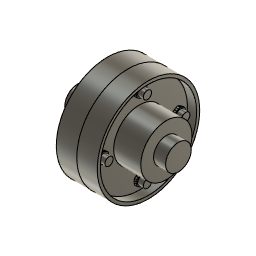
Sketch31_Final v1 (Autodesk Fusion 360 design; units mm, degrees)
Autodesk Fusion 360 part; units mm, degrees
sketch "Sketch1" plane through (0, 0, 0) normal (0, 1, 0) x (1, 0, 0)
  line L0 (0, -25) -> (0, -45)
  line L1 (0, -25) -> (0, -100)
  line L2 (0, -100) -> (40, -100)
  line L3 (40, -100) -> (40, -94)
  line L4 (0, -100) -> (22, -100)
  line L5 (22, -100) -> (22, -94)
  line L6 (22, -94) -> (0, -94)
  line L7 (40, -94) -> (22, -94)
  line L8 (0, -25) -> (0, -50)
  line L9 (22, -94) -> (22, -50)
  line L10 (0, -50) -> (22, -50)
  line L11 (75, -25) -> (75, -50)
  line L12 (22, -50) -> (75, -50)
  line L13 (0, -45) -> (-5, -45)
  line L14 (-5, -45) -> (-5, -25)
  line L15 (0, -25) -> (-5, -25)
  line L16 (0, -25) -> (75, -25)
  dimension "d3" = 45
  dimension "d4" = 100
  dimension "d5" = 40
  dimension "d6" = 6
  dimension "d9" = 25
  dimension "d10" = 50
  dimension "d12" = 5
  constraint vertical L0
  constraint parallel L0 L1
  constraint perpendicular L1 L2
  constraint perpendicular L2 L3
  constraint perpendicular L1 L4
  constraint perpendicular L4 L5
  constraint coincident L1 L6.end
  constraint perpendicular L1 L6
  constraint perpendicular L6 L9
  constraint perpendicular L9 L10
  constraint perpendicular L11 L12
  constraint perpendicular L8 L13
  constraint perpendicular L13 L14
  constraint perpendicular L14 L15
  measures "d3" distance of origin L0.end
  measures "d4" distance of origin L1.end
  measures "d5" distance of L1.end L2.end
  measures "d6" distance of L2.end L3.end
  measures "d9" distance of origin L0.start
  measures "d10" distance of origin L8.end
  measures "d12" distance of L0.end L13.end
revolve "Revolve1" add sketch "Sketch1" angle 360 about axis through (1.75, 0, 0) along (1, 0, 0) makes body 1
hole "Hole1" at (0, -2.3677, 72.2147) direction (1, 0, 0) diameter 16 depth 70 tip angle 118 bodies 1
pattern_circular "C-Pattern1" count 4 over 360 about axis through (1.75, 0, 0) along (1, 0, 0) of "Hole1"
copy_body "Body->Comp1" bodies 1 removing the originals makes body 2 in component "Male Flange"
sketch "Sketch2" plane through (0, 0, 0) normal (0, 1, 0) x (1, 0, 0)
  line L0 (5, -25) -> (75, -25)
  line L1 (75, -25) -> (75, -50)
  line L2 (75, -50) -> (0, -50)
  line L3 (0, -50) -> (0, -100)
  line L4 (0, -100) -> (40, -100)
  line L5 (40, -100) -> (40, -94)
  line L6 (40, -94) -> (22, -94)
  line L7 (22, -94) -> (22, -50)
  line L8 (0, -50) -> (0, -45)
  line L9 (5, -25) -> (5, -45)
  line L10 (5, -45) -> (0, -45)
  constraint horizontal L0
  constraint perpendicular L0 L1
  constraint perpendicular L1 L2
  constraint perpendicular L0 L3
  constraint perpendicular L3 L4
  constraint perpendicular L4 L5
  constraint perpendicular L5 L6
  constraint coincident L2 L7.end
  constraint perpendicular L2 L7
  constraint perpendicular L0 L8
  constraint perpendicular L0 L9
  constraint perpendicular L8 L10
revolve "Revolve2" add sketch "Sketch2" angle 360 about axis through (1.75, 0, 0) along (1, 0, 0) separate body makes body 3
hole "Hole2" at (0, 10.3242, 67.7446) direction (1, 0, 0) diameter 16 depth 70 tip angle 118 bodies 3
pattern_circular "C-Pattern2" count 4 over 360 about axis through (1.75, 0, 0) along (1, 0, 0) of "Hole2"
copy_body "Body->Comp2" bodies 3 removing the originals makes body 4 in component "Female Flange"
sketch "Sketch3" plane through (0, 0, 0) normal (1, 0, 0) x (0, 1, 0)
  circle A0 centre (0, 0) radius 25
  dimension "d26" = 50
  constraint coincident A0.centre origin
  measures "d26" diameter of A0
extrude "Extrude1" add sketch "Sketch3" along normal blind 100 separate body makes body 5
copy_body "Body->Comp3" bodies 5 removing the originals makes body 6 in component "Shaft"
sketch "Sketch4" plane through (0, 0, 0) normal (0, 1, 0) x (1, 0, 0)
  line L0 (0, 0) -> (0, -8)
  line L1 (0, -8) -> (44, -8)
  line L2 (44, -8) -> (44, 0)
  line L3 (44, 0) -> (0, 0)
  line L4 (0, 0) -> (0, -16)
  line L5 (0, -16) -> (-16, -16)
  line L6 (-16, -16) -> (-16, 0)
  line L7 (-16, 0) -> (0, 0)
  line L8 (0, -8) -> (60, -8)
  line L9 (60, -8) -> (60, 0)
  line L10 (60, 0) -> (44, 0)
  dimension "d29" = 8
  dimension "d30" = 44
  dimension "d31" = 16
  dimension "d32" = 16
  dimension "d33" = 60
  constraint coincident L0.start L3.end
  constraint vertical L0
  constraint perpendicular L0 L1
  constraint perpendicular L1 L2
  constraint perpendicular L0 L3
  constraint perpendicular L1 L4
  constraint perpendicular L4 L5
  constraint perpendicular L5 L6
  constraint perpendicular L0 L7
  constraint perpendicular L2 L8
  constraint perpendicular L8 L9
  constraint perpendicular L2 L10
  measures "d29" distance of L0.start L0.end
  measures "d30" distance of L0.end L1.end
  measures "d31" distance of L0.start L4.end
  measures "d32" distance of L4.end L5.end
  measures "d33" distance of L0.end L8.end
revolve "Revolve3" add sketch "Sketch4" angle 360 about axis through (1.75, 0, 0) along (1, 0, 0) separate body makes body 7
copy_body "Body->Comp4" bodies 7 removing the originals makes body 8 in component "Nut"
delete_face "DeleteFace1" 1 faces at (7.3333, 10.7229, 75.7346) on bodies 4 in component "Female Flange"
delete_face "DeleteFace2" 1 faces at (7.3333, -75.7346, 10.7229) on bodies 4 in component "Female Flange"
delete_face "DeleteFace3" 1 faces at (7.3333, -10.7229, -75.7346) on bodies 4 in component "Female Flange"
delete_face "DeleteFace4" 1 faces at (7.3333, 75.7346, -10.7229) on bodies 4 in component "Female Flange"
sketch "Sketch5" plane through (26.2431, 112.1215, 282.1453) normal (1, 0, 0) x (0, 1, 0)
  circle A0 centre (0, 0) radius 75
  line L0 (0, 0) -> (0, 100)
  circle A1 centre (0, 75) radius 8
  circle A2 centre (-75, 0) radius 8
  circle A3 centre (0, -75) radius 8
  circle A4 centre (75, 0) radius 8
  dimension "d35" = 16
  dimension "d37" = 360
  constraint coincident A0.centre L0.start
  constraint vertical L0
  constraint coincident A0 A1.centre
  constraint coincident L0 A1.centre
  measures "d35" diameter of A1
extrude "Extrude1'" cut sketch "Sketch5" along normal blind 40 contours A0 A4 | A0 A4 | A0 L0 A1 | A0 L0 A1 | A0 A3 | A0 A3 | A0 L0 A1 | A0 L0 A1 | A0 A2 | A0 A2 sketch seen with x (1, 0, 0) y (0, 1, 0) z (0, 0, 1) at (-26.2431, -112.1215, -282.1453) bodies 4 in component "Female Flange"
delete_face "DeleteFace1'" 1 faces at (14.6667, -1.5711, 80.1749) on bodies 2 in component "Male Flange"
delete_face "DeleteFace2'" 1 faces at (14.6667, 80.1749, 1.5711) on bodies 2 in component "Male Flange"
delete_face "DeleteFace3'" 1 faces at (14.6667, -80.1749, -1.5711) on bodies 2 in component "Male Flange"
delete_face "DeleteFace4'" 1 faces at (14.6667, 1.5711, -80.1749) on bodies 2 in component "Male Flange"
sketch "Sketch6" plane through (244.9205, 122.5963, 325.0714) normal (1, 0, 0) x (0, 1, 0)
  circle A0 centre (0, 0) radius 75
  line L0 (0, 0) -> (0, 75)
  circle A1 centre (0, 75) radius 8
  circle A2 centre (-75, 0) radius 8
  circle A3 centre (0, -75) radius 8
  circle A4 centre (75, 0) radius 8
  dimension "d40" = 150
  dimension "d41" = 16
  dimension "d43" = 360
  constraint coincident A0.centre L0.start
  constraint coincident A0 L0.end
  constraint vertical L0
  constraint coincident L0.end A1.centre
  measures "d40" diameter of A0
  measures "d41" diameter of A1
extrude "Extrude1''" cut sketch "Sketch6" along normal blind 30 contours A0 A4 | A0 A4 | A0 L0 A1 | A0 A1 | A0 A3 | A0 A3 | A0 L0 A1 | A0 A2 | A0 A2 sketch seen with x (1, 0, 0) y (0, 1, 0) z (0, 0, 1) at (-244.9205, -122.5963, -325.0714) bodies 2 in component "Male Flange"
sketch "Sketch7" plane through (0, 0, 0) normal (1, 0, 0) x (0, 1, 0)
  circle A0 centre (0, 0) radius 8
  circle A1 centre (0, 0) radius 10
  arc A2 (0, 11) -> (3.311, 9.436) centre (111.0644, 241.8306) ccw
  arc A3 (-3.311, 9.436) -> (0, 11) centre (-111.0644, 241.8306) ccw
  arc A4 (-9.5263, 5.5) -> (-6.5163, 7.5854) centre (-153.8992, 217.0999) ccw
  arc A5 (-9.8273, 1.8506) -> (-9.5263, 5.5) centre (-264.9636, 24.7307) ccw
  arc A6 (-9.5263, -5.5) -> (-9.8273, -1.8506) centre (-264.9636, -24.7307) ccw
  arc A7 (-6.5163, -7.5854) -> (-9.5263, -5.5) centre (-153.8992, -217.0999) ccw
  arc A8 (0, -11) -> (-3.311, -9.436) centre (-111.0644, -241.8306) ccw
  arc A9 (3.311, -9.436) -> (0, -11) centre (111.0644, -241.8306) ccw
  arc A10 (9.5263, -5.5) -> (6.5163, -7.5854) centre (153.8992, -217.0999) ccw
  arc A11 (9.8273, -1.8506) -> (9.5263, -5.5) centre (264.9636, -24.7307) ccw
  arc A12 (9.5263, 5.5) -> (9.8273, 1.8506) centre (264.9636, 24.7307) ccw
  arc A13 (6.5163, 7.5854) -> (9.5263, 5.5) centre (153.8992, 217.0999) ccw
  dimension "d74" = 16
  dimension "d75" = 20
  dimension "d80" = 360
  constraint coincident A0.centre A1.centre
  constraint concentric A0 A1
  constraint coincident A1 A2.end
  measures "d74" diameter of A0
  measures "d75" diameter of A1
extrude "Extrude2" add sketch "Sketch7" along normal blind 5 separate body makes body 9
copy_body "Body->Comp5" bodies 9 removing the originals makes body 10 in component "Bolt"
component "Male Flange" placed x (-1, 0, 0) y (0, -1, 0) z (0, 0, 1) at (140.7245, 338.6063, 122.8818)
component "Female Flange" placed x (1, 0, 0) y (0, 1, 0) z (0, 0, 1) at (140.7245, 338.6063, 122.8818)
component "Shaft" placed x (1, 0, 0) y (0, 1, 0) z (0, 0, 1) at (139.2245, 338.6063, 122.8818)
component "Shaft" placed x (1, 0, 0) y (0, 1, 0) z (0, 0, 1) at (42.2245, 338.6063, 122.8818)
component "Nut" placed x (1, 0, 0) y (0, 1, 0) z (0, 0, 1) at (118.7245, 338.6063, 47.8818)
component "Nut" placed x (1, 0, 0) y (0, 1, 0) z (0, 0, 1) at (118.7245, 263.6063, 122.8818)
component "Nut" placed x (1, 0, 0) y (0, 1, 0) z (0, 0, 1) at (118.7245, 338.6063, 197.8818)
component "Nut" placed x (1, 0, 0) y (0, 1, 0) z (0, 0, 1) at (118.7245, 413.6063, 122.8818)
component "Bolt" placed x (1, 0, 0) y (0, 1, 0) z (0, 0, 1) at (162.7245, 338.6063, 197.8818)
component "Bolt" placed x (1, 0, 0) y (0, 1, 0) z (0, 0, 1) at (162.7245, 413.6063, 122.8818)
component "Bolt" placed x (-1, 0, 0) y (0, -1, 0) z (0, 0, 1) at (167.7245, 263.6063, 122.8818)
component "Bolt" placed x (-1, 0, 0) y (0, -1, 0) z (0, 0, 1) at (167.7245, 338.6063, 47.8818)
named bodies: "Male Flange", "Female Flange", "Shaft", "Nut", "Bolt"
